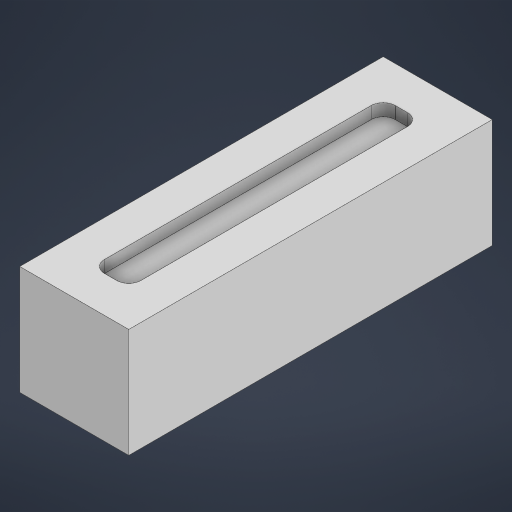
# Autodesk Inventor part: oled_support
Saved by Autodesk Inventor 2024.2 (Build 282272000, 272)
## iProperties
Created: 2024-09-18
Part Number: oled_support
Material: Generic
Document SubType Name: Modeling
Designer: Moe
Density: 1 g/cm^3
Appearance: Default
Author: Moe
Autodesk Inventor part; units mm, degrees
ref_plane "YZ Plane" through (0, 0, 0) normal (1, 0, 0) x (0, 1, 0)
ref_plane "XZ Plane" through (0, 0, 0) normal (0, 1, 0) x (-1, 0, 0)
ref_plane "XY Plane" through (0, 0, 0) normal (0, 0, 1) x (1, 0, 0)
sketch "Sketch1" plane through (0, 0, 0) normal (0, 1, 0) x (-1, 0, 0)
  line L0 (0, 0) -> (9, 0)
  line L1 (9, 0) -> (9, -30)
  line L2 (9, -30) -> (0, -30)
  line L3 (0, -30) -> (0, 0)
  dimension "d0" = 9
  dimension "d1" = 30
  constraints: 8 end point, 2 parallel, 1 horizontal, 1 perpendicular
  measures "d0" distance of L1.end L2.end
  measures "d1" distance of L0.end L1.end
extrude "Extrusion1" add sketch "Sketch1" along normal blind 9
sketch "Sketch2" plane through (0, 0, 0) normal (0, -1, 0) x (1, 0, 0)
  line L0 (-3, -3) -> (-6, -3)
  line L1 (-6, -3) -> (-6, -27)
  line L2 (-6, -27) -> (-3, -27)
  line L3 (-3, -27) -> (-3, -3)
  line L4 (0, 0) -> (0, -30) projected
  line L5 (-9, -30) -> (-9, 0) projected
  line L6 (-9, 0) -> (0, 0) projected
  line L7 (0, -30) -> (-9, -30) projected
  point P0 (-4.5, 0)
  point P1 (-4.5, -30)
  dimension "d4" = 3
  dimension "d5" = 3
  dimension "d6" = 3
  dimension "d7" = 3
  constraints: 8 end point, 2 midpoint, 2 parallel, 1 horizontal, 1 perpendicular
  measures "d4" distance between parallel lines of L4 L3
  measures "d5" distance between parallel lines of L5 L1
  measures "d6" distance from line of point (-4.5, 0) L0
  measures "d7" distance from line of point (-4.5, -30) L2
extrude "Extrusion2" cut sketch "Sketch2" against normal blind 1 contours L3 L2 L1 L0
fillet "Fillet1" radius 1 4 edges at (-6, 0.5, -27) (-3, 0.5, -27) (-6, 0.5, -3) (-3, 0.5, -3)
sketch "Sketch3" plane through (0, 9, 0) normal (0, 1, 0) x (1, 0, 0)
  line L0 (-5, 3) -> (-4, 3)
  line L1 (-3, 4) -> (-3, 26)
  line L2 (-4, 27) -> (-5, 27)
  line L3 (-6, 26) -> (-6, 4)
  arc A0 (-6, 4) -> (-5, 3) centre (-5, 4) ccw
  arc A1 (-5, 27) -> (-6, 26) centre (-5, 26) ccw
  arc A2 (-3, 26) -> (-4, 27) centre (-4, 26) ccw
  arc A3 (-4, 3) -> (-3, 4) centre (-4, 4) ccw
  line L4 (0, 0) -> (0, 30) projected
  line L5 (-9, 30) -> (-9, 0) projected
  line L6 (-9, 0) -> (0, 0) projected
  line L7 (0, 30) -> (-9, 30) projected
  point P0 (-4.5, 0)
  point P1 (-4.5, 3)
  point P2 (-4.5, 30)
  point P3 (-4.5, 27)
  dimension "d11" = 1
  dimension "d12" = 1
  dimension "d13" = 3
  dimension "d14" = 3
  dimension "d15" = 3
  dimension "d16" = 3
  constraints: 8 end point, 8 point on circle, 8 tangent, 4 centre point, 4 midpoint, 2 equal radius, 2 parallel, 1 horizontal, 1 perpendicular
  measures "d11" radius of A0
  measures "d12" radius of A1
  measures "d13" distance between parallel lines of L4 L1
  measures "d14" distance between parallel lines of L5 L3
  measures "d15" distance of point (-4.5, 0) point (-4.5, 3)
  measures "d16" distance of point (-4.5, 30) point (-4.5, 27)
extrude "Extrusion3" cut sketch "Sketch3" against normal blind 1 contours A0 L3 A1 L2 A2 L1 A3 L0
body "Solid1"
